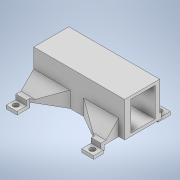
# Autodesk Inventor part: U2D2 Plate v2
Saved by Autodesk Inventor 2022 (Build 260153000, 153)
## iProperties
Created: 2021-09-20
Part Number: U2D2 Plate v2
Material: Generic
Document SubType Name: Modeling
Designer: kylem
Density: 1 g/cm^3
Appearance: Default
Author: kylem
Autodesk Inventor part; units mm, degrees
note: some values were not read from the file. Chosen so that the rebuilt part matches the saved one: edges of "Chamfer23".
ref_plane "YZ Plane" through (0, 0, 0) normal (1, 0, 0) x (0, 1, 0)
sketch "Sketch1" plane through (0, 0, 0) normal (0, 1, 0) x (-1, 0, 0)
  line L0 (0, 0) -> (3, 0)
  line L1 (3, 0) -> (3, -3)
  line L2 (0, 0) -> (-48.04, 0)
  line L3 (-48.04, 0) -> (-54, 0)
  line L4 (3, -3) -> (-54, -3)
  line L5 (-54, -3) -> (-54, 45)
  line L6 (-54, 45) -> (3, 45)
  line L7 (3, 45) -> (3, -3)
  line L8 (3, 21) -> (6.1215, 21)
  circle A0 centre (0, 0) radius 1.65
  circle A1 centre (-48.04, 0) radius 1.65
  line L9 (0, 42) -> (-48.04, 42)
  circle A2 centre (0, 42) radius 1.65
  circle A3 centre (-48.04, 42) radius 1.65
  line L10 (-54, -3) -> (-54, 8.785)
  line L11 (-54, 8.785) -> (-9.9, 8.785)
  line L12 (-9.9, 8.785) -> (-9.9, 23.785)
  line L13 (-9.9, 23.785) -> (-54, 23.785)
  dimension "d0" = 3
  dimension "d1" = 3
  dimension "d2" = 48.04
  dimension "d3" = 5.96
  dimension "d4" = 48
  dimension "d5" = 3.3
  dimension "d6" = 3.3
  dimension "d7" = 11.785
  dimension "d8" = 44.1
  dimension "d9" = 15
  constraints: 28 end point, 5 perpendicular, 4 centre point, 4 coincident, 4 horizontal, 4 symmetric about line, 3 point on line, 2 parallel, 1 midpoint, 2 other
  measures "d0" distance of L0.start L0.end
  measures "d1" distance of L0.end L1.end
  measures "d2" distance of L0.start L2.end
  measures "d3" distance of L2.end L3.end
  measures "d4" distance of L4.end L5.end
  measures "d5" diameter of A0
  measures "d6" diameter of A1
  measures "d7" distance of L4.end L10.end
  measures "d8" distance of L10.end L11.end
  measures "d9" distance of L11.end L12.end
extrude "Extrusion1" add sketch "Sketch1" along normal blind 2 contours A0 L2 A1 L3 L5 L11 L12 L13 L6 L7 L0 | L0 L1 L4 L5 L3 A1 L2 A0
sketch "Sketch2" plane through (0, 0, 0) normal (0, -1, 0) x (1, 0, 0)
  line L0 (-3, -3) -> (-3, 45) projected
  line L1 (-3, -3) -> (-3, 5)
  line L2 (54, 8.785) -> (54, -3) projected
  line L3 (9.9, 8.785) -> (54, 8.785) projected
  line L4 (54, 8.785) -> (54, 4.785)
  line L5 (54, 8.785) -> (54, -3) projected
  line L6 (54, 23.785) -> (54, 27.785)
  line L7 (54, 45) -> (54, 23.785) projected
  line L8 (54, 27.785) -> (-3, 27.785)
  line L9 (-3, 5) -> (-3, 27.785)
  line L10 (9.9, 8.785) -> (54, 8.785) projected
  line L11 (54, 8.785) -> (9.9, 8.785)
  line L12 (9.9, 23.785) -> (9.9, 8.785) projected
  line L13 (9.9, 8.785) -> (9.9, 23.785)
  line L14 (9.9, 23.785) -> (54, 23.785)
  line L15 (-3, 5) -> (-3, 27.785)
  line L16 (-3, 27.785) -> (54, 27.785)
  line L17 (54, 27.785) -> (54, 4.785)
  line L18 (54, 4.785) -> (-3, 4.785)
  line L19 (-3, 4.785) -> (-3, 27.785)
  point P0 (0, 0)
  point P1 (-3, 4.785)
  dimension "d12" = 8
  dimension "d13" = 4
  dimension "d14" = 4
  constraints: 26 end point, 4 collinear, 4 point on line, 3 perpendicular, 2 parallel, 1 horizontal
  measures "d12" distance of L0.start L1.end
  measures "d13" distance of L2.start L4.end
  measures "d14" distance of L6.start L6.end
ref_plane "Work Plane1" through (0, -7, 0) normal (0, -1, 0) x (1, 0, 0)
sketch "Sketch4" plane through (54, 0, -3) normal (1, 0, 0) x (0, 0, -1)
  line L0 (-7.785, 0) -> (-7.785, -7) projected
  line L1 (-7.785, 0) -> (-7.785, 2)
  line L2 (0, 2) -> (-48, 2) projected
  line L3 (-7.785, 2) -> (-7.785, 15)
  line L4 (-30.785, 0) -> (-30.785, -7) projected
  line L5 (-30.785, 0) -> (-30.785, 15)
  line L6 (-7.785, 15) -> (-30.785, 15)
  line L7 (-26.785, -5) -> (-11.785, -5) projected
  line L8 (-11.785, 0) -> (-11.785, 2) projected
  line L9 (-11.785, -5) -> (-11.785, 2)
  line L10 (-11.785, 2) -> (-11.785, 13)
  line L11 (-26.785, 0) -> (-26.785, 2) projected
  line L12 (-26.785, 2) -> (-26.785, 13)
  line L13 (-26.785, 13) -> (-11.785, 13)
  point P0 (-3, 0)
  point P1 (-30.785, 2)
  dimension "d19" = 13
  dimension "d20" = 15
  dimension "d21" = 11
  dimension "d22" = 11
  constraints: 16 end point, 3 point on line, 2 collinear, 2 vertical
  measures "d19" distance of L1.end L3.end
  measures "d20" distance of L4.start L5.end
  measures "d21" distance of L8.end L10.end
  measures "d22" distance of L11.end L12.end
extrude "Extrusion5" add sketch "Sketch2" along normal blind 7 contours L0 L8 L6 L14 L12 L3 L2 L18
sketch "Sketch5" plane through (0, -7, 0) normal (0, -1, 0) x (1, 0, 0)
  line L0 (9.9, 23.785) -> (54, 23.785) projected
  line L1 (54, 23.785) -> (9.9, 23.785)
  line L2 (9.9, 23.785) -> (9.9, 8.785)
  line L3 (9.9, 8.785) -> (54, 8.785)
  line L4 (54, 8.785) -> (54, 23.785)
  point P0 (0, 0)
  constraints: 8 end point, 2 parallel, 1 horizontal, 1 perpendicular
extrude "Extrusion6" add sketch "Sketch5" against normal blind 2
extrude "Extrusion7" add sketch "Sketch4" against normal blind 44.1 contours L2 L10 L13 L12 L5 L6 L3
sketch "Sketch6" plane through (9.9, 0, -3) normal (-1, 0, 0) x (0, 0, 1)
  line L0 (7.785, 15) -> (7.785, 2) projected
  line L1 (48, 2) -> (30.785, 2) projected
  line L2 (7.785, 15) -> (30.785, 15)
  line L3 (30.785, 15) -> (30.785, 2)
  line L4 (30.785, 2) -> (7.785, 2)
  line L5 (7.785, 2) -> (7.785, 15)
  point P0 (3, 0)
  constraints: 8 end point, 2 parallel, 1 horizontal, 1 perpendicular
extrude "Extrusion8" add sketch "Sketch6" along normal blind 12.9
sketch "Sketch8" plane through (9.9, -5, 8.785) normal (0, 0, 1) x (1, 0, 0)
  line L0 (44.1, 0) -> (44.1, 18) projected
  line L1 (44.1, 0) -> (18.5, 0)
  line L2 (0, 0) -> (44.1, 0) projected
  line L3 (18.5, 0) -> (5.5, 0)
  line L4 (5.5, 0) -> (5.5, 1)
  line L5 (-12.9, 5) -> (44.1, 5) projected
  line L6 (5.5, 1) -> (14.6, 1)
  line L7 (44.1, -2) -> (-12.9, -2) projected
  line L8 (44.1, 18) -> (0, 18) projected
  line L9 (14.6, -2) -> (36.6, -2) construction
  line L10 (5.5, 1) -> (5.5, 18)
  line L11 (5.5, 18) -> (14.6, 18)
  line L12 (44.1, 18) -> (0, 18) projected
  line L13 (5.5, 1) -> (5.5, 17)
  line L14 (5.5, 17) -> (14.6, 17)
  line L15 (5.5, 17) -> (18.5, 17)
  line L16 (18.5, 17) -> (18.5, 1)
  line L17 (18.5, 1) -> (5.5, 1)
  point P0 (-9.9, 5)
  point P1 (5.5, 5)
  point P2 (14.6, 1)
  dimension "d33" = 25.6
  dimension "d34" = 13
  dimension "d35" = 1
  dimension "d39" = 16
  dimension "d42" = 13
  constraints: 24 end point, 7 point on line, 3 perpendicular, 1 collinear, 1 horizontal
  measures "d33" distance of L0.start L1.end
  measures "d34" distance of L1.end L3.end
  measures "d35" distance of L3.end L4.end
  measures "d39" distance of L4.end L13.end
  measures "d42" distance of L13.end L15.end
extrude "Extrusion10" cut sketch "Sketch8" against normal blind 12.9 contours L16 L17 L6 L10 L5 | L5 L10 L14 L15 L16
sketch "Sketch11" plane through (0, 2, 0) normal (0, 1, 0) x (1, 0, 0)
  circle A0 centre (48.04, 0) radius 1.65 projected
  circle A1 centre (0, 0) radius 1.65 projected
  line L0 (48.04, 0) -> (0, 0)
  line L1 (24.02, 0) -> (24.02, 5.2317)
  line L2 (24.02, 0) -> (10.02, 0)
  line L3 (10.02, 0) -> (38.02, 0)
  line L4 (38.02, 0) -> (38.02, 7.5339)
  line L5 (54, -4.785) -> (-3, -4.785) projected
  line L6 (38.02, 7.5339) -> (10.02, 7.5339)
  line L7 (10.02, 7.5339) -> (10.02, -4.785)
  line L8 (10.02, -4.785) -> (38.02, -4.785)
  line L9 (38.02, -4.785) -> (38.02, 7.5339)
  dimension "d74" = 14
  dimension "d75" = 28
  constraints: 18 end point, 3 point on line, 2 horizontal, 2 parallel, 2 perpendicular, 1 midpoint, 1 vertical
  measures "d74" distance of L1.start L2.end
  measures "d75" distance of L2.end L3.end
extrude "Extrusion12" cut sketch "Sketch11" against normal blind 10 contours L9 L5 L7 L0 | L0 L7 L6 L4
chamfer "Chamfer9" distance 7.785 angle 45 2 edges at (38.02, 1, -3) (10.02, 1, -3)
sketch "Sketch12" plane through (54, 13, 8.785) normal (0, -1, 0) x (1, 0, 0)
  line L0 (0, 0) -> (-44.1, 0) projected
  line L1 (-44.1, 0) -> (-44.1, 15) projected
  line L2 (0, 0) -> (-44.1, 0)
  line L3 (-44.1, 0) -> (-44.1, 15)
  line L4 (-44.1, 15) -> (0, 15)
  line L5 (0, 15) -> (0, 0)
  point P0 (-54, -8.785)
  constraints: 8 end point, 2 parallel, 1 horizontal, 1 perpendicular
extrude "Extrusion13" cut sketch "Sketch12" against normal blind 0.17
sketch "Sketch13" plane through (0, -5, 0) normal (0, 1, 0) x (1, 0, 0)
  line L0 (54, -23.785) -> (9.9, -23.785) projected
  line L1 (9.9, -8.785) -> (54, -8.785)
  line L2 (54, -8.785) -> (54, -23.785)
  line L3 (54, -23.785) -> (9.9, -23.785)
  line L4 (9.9, -23.785) -> (9.9, -8.785)
  point P0 (0, 0)
  constraints: 8 end point, 2 parallel, 1 horizontal, 1 perpendicular
extrude "Extrusion14" cut sketch "Sketch13" against normal blind 0.17
sketch "Sketch14" plane through (54, 13.17, 23.785) normal (0, 0, -1) x (-1, 0, 0)
  line L0 (44.1, -18.34) -> (44.1, 0) projected
  line L1 (0, -18.34) -> (44.1, -18.34) projected
  line L2 (44.1, 0) -> (0, 0)
  line L3 (0, 0) -> (0, -18.34)
  line L4 (0, -18.34) -> (44.1, -18.34)
  line L5 (44.1, -18.34) -> (44.1, 0)
  point P0 (54, -13.17)
  constraints: 8 end point, 2 parallel, 1 horizontal, 1 perpendicular
extrude "Extrusion15" cut sketch "Sketch14" against normal blind 0.07
sketch "Sketch15" plane through (9.9, 13.17, 8.785) normal (0, 0, 1) x (1, 0, 0)
  line L0 (44.1, 0) -> (0, 0) projected
  line L1 (44.1, 0) -> (44.1, -18.34) projected
  line L2 (0, 0) -> (44.1, 0)
  line L3 (44.1, 0) -> (44.1, -18.34)
  line L4 (44.1, -18.34) -> (0, -18.34)
  line L5 (0, -18.34) -> (0, 0)
  point P0 (-9.9, -13.17)
  constraints: 8 end point, 2 parallel, 1 horizontal, 1 perpendicular
extrude "Extrusion16" cut sketch "Sketch15" against normal blind 0.07
ref_plane "Work Plane2" through (0, -10, 0) normal (0, -1, 0) x (1, 0, 0)
sketch "Sketch16" plane through (0, -10, 0) normal (0, -1, 0) x (1, 0, 0)
  circle A0 centre (0, 42) radius 1.65 projected
  circle A1 centre (0, 42) radius 1.65
  line L0 (0, 42) -> (0, 45)
  line L1 (-3, 45) -> (54, 45) projected
  line L2 (0, 45) -> (3.75, 45)
  line L3 (3.75, 45) -> (3.75, 39)
  line L4 (3.75, 39) -> (-3.75, 39)
  line L5 (-3.75, 39) -> (-3.75, 45)
  line L6 (-3.75, 45) -> (3.75, 45)
  circle A2 centre (48.04, 42) radius 1.65 projected
  line L7 (0, 42) -> (48.04, 42)
  line L8 (24.02, 42) -> (24.02, 49.286)
  circle A3 centre (48.04, 42) radius 1.65
  circle A4 centre (48.04, 42) radius 1.65
  line L9 (48.04, 42) -> (48.04, 45)
  line L10 (51.04, 45) -> (-5.96, 45)
  line L11 (48.04, 45) -> (44.29, 45)
  line L12 (44.29, 45) -> (44.29, 39)
  line L13 (44.29, 39) -> (51.79, 39)
  line L14 (51.79, 39) -> (51.79, 45)
  line L15 (51.79, 45) -> (44.29, 45)
  line L16 (48.04, 42) -> (0, 42)
  line L17 (0, 42) -> (0, 0)
  line L18 (0, 21) -> (5.7249, 21)
  circle A5 centre (0, 0) radius 1.65
  circle A6 centre (0, 0) radius 1.65
  line L19 (0, 0) -> (0, -3)
  line L20 (-3, -3) -> (54, -3)
  line L21 (0, -3) -> (3.75, -3)
  line L22 (3.75, -3) -> (3.75, 3)
  line L23 (3.75, 3) -> (-3.75, 3)
  line L24 (-3.75, 3) -> (-3.75, -3)
  line L25 (-3.75, -3) -> (3.75, -3)
  circle A7 centre (48.04, 0) radius 1.65
  line L26 (0, 0) -> (48.04, 0)
  line L27 (24.02, 0) -> (24.02, -7.286)
  circle A8 centre (48.04, 0) radius 1.65
  circle A9 centre (48.04, 0) radius 1.65
  line L28 (48.04, 0) -> (48.04, -3)
  line L29 (51.04, -3) -> (-5.96, -3)
  line L30 (48.04, -3) -> (44.29, -3)
  line L31 (44.29, -3) -> (44.29, 3)
  line L32 (44.29, 3) -> (51.79, 3)
  line L33 (51.79, 3) -> (51.79, -3)
  line L34 (51.79, -3) -> (44.29, -3)
  line L35 (48.04, 0) -> (0, 0)
  line L36 (0, 0) -> (0, 42)
  line L37 (44.29, 39) -> (50.29, 39)
  line L38 (50.29, 39) -> (50.29, 37)
  line L39 (50.29, 37) -> (44.29, 37)
  line L40 (44.29, 37) -> (44.29, 39)
  line L41 (3.75, 39) -> (-3.75, 39)
  line L42 (-3.75, 39) -> (-3.75, 37)
  line L43 (-3.75, 37) -> (3.75, 37)
  line L44 (3.75, 37) -> (3.75, 39)
  line L45 (3.75, 3) -> (-3.75, 3)
  line L46 (-3.75, 3) -> (-3.75, 4.785)
  line L47 (-3.75, 4.785) -> (3.75, 4.785)
  line L48 (3.75, 4.785) -> (3.75, 3)
  line L49 (-3, 4.785) -> (54, 4.785) projected
  line L50 (51.79, 3) -> (44.29, 3)
  line L51 (44.29, 3) -> (44.29, 4.785)
  line L52 (44.29, 4.785) -> (51.79, 4.785)
  line L53 (51.79, 4.785) -> (51.79, 3)
  dimension "d102" = 3.75
  dimension "d103" = 6
  dimension "d104" = 7.5
  dimension "d107" = 6
  dimension "d108" = 2
  dimension "d109" = 2
  constraints: 104 end point, 33 symmetric about line, 9 perpendicular, 8 centre point, 8 parallel, 7 point on line, 6 horizontal, 4 coincident, 2 midpoint, 2 vertical, 1 collinear, 7 other
  measures "d102" distance of L0.end L2.end
  measures "d103" distance of L2.end L3.end
  measures "d104" distance of L3.end L4.end
  measures "d107" distance of L38.end L39.end
  measures "d108" distance of L37.end L38.end
  measures "d109" distance of L42.end L41.end
extrude "Extrusion18" add sketch "Sketch16" against normal blind 2 contours L7 L3 L4 L17 A0 | A0 L0 L1 L3 L7 | A0 L17 L4 L5 L6 L1 L0 | L17 L43 L42 L4 | L4 L44 L43 L17 | L12 L1 L9 A2 L7 | L7 A2 L9 L1 L14 L13 L12 | L13 L38 L39 L40 | L47 L48 L23 L17 | L17 L23 L46 L47 | L23 L22 L26 A5 L17 | L17 A5 L19 L20 L25 L24 L23 | L49 L53 L32 L51 | L26 L22 L20 L19 A5 | L32 L33 L20 L28 A7 L26 L31 | L26 A7 L28 L20 L31
sketch "Sketch19" plane through (0, -10, 0) normal (0, -1, 0) x (1, 0, 0)
  circle A0 centre (0, 42) radius 1.65
  circle A1 centre (0, 42) radius 1.65
  line L0 (0, 42) -> (0, 45)
  line L1 (-3, 45) -> (54, 45)
  line L2 (0, 45) -> (3.75, 45)
  line L3 (3.75, 45) -> (3.75, 39)
  line L4 (3.75, 39) -> (-3.75, 39)
  line L5 (-3.75, 39) -> (-3.75, 45)
  line L6 (-3.75, 45) -> (3.75, 45)
  circle A2 centre (48.04, 42) radius 1.65
  line L7 (0, 42) -> (48.04, 42)
  line L8 (24.02, 42) -> (24.02, 49.286)
  circle A3 centre (48.04, 42) radius 1.65
  circle A4 centre (48.04, 42) radius 1.65
  line L9 (48.04, 42) -> (48.04, 45)
  line L10 (51.04, 45) -> (-5.96, 45)
  line L11 (48.04, 45) -> (44.29, 45)
  line L12 (44.29, 45) -> (44.29, 39)
  line L13 (44.29, 39) -> (51.79, 39)
  line L14 (51.79, 39) -> (51.79, 45)
  line L15 (51.79, 45) -> (44.29, 45)
  line L16 (48.04, 42) -> (0, 42)
  line L17 (0, 42) -> (0, 0)
  line L18 (0, 21) -> (5.7249, 21)
  circle A5 centre (0, 0) radius 1.65
  circle A6 centre (0, 0) radius 1.65
  line L19 (0, 0) -> (0, -3)
  line L20 (0, -3) -> (3.75, -3)
  line L21 (3.75, -3) -> (3.75, 3)
  line L22 (3.75, 3) -> (-3.75, 3)
  line L23 (-3.75, 3) -> (-3.75, -3)
  line L24 (-3.75, -3) -> (3.75, -3)
  line L25 (0, 0) -> (0, 42)
  line L26 (-3, -3) -> (54, -3)
  line L27 (24.02, 0) -> (24.02, -7.286)
  line L28 (44.29, -3) -> (44.29, 3)
  line L29 (48.04, -3) -> (44.29, -3)
  line L30 (0, 0) -> (48.04, 0)
  line L31 (48.04, 0) -> (48.04, -3)
  line L32 (48.04, 0) -> (0, 0)
  circle A7 centre (48.04, 0) radius 1.65
  circle A8 centre (48.04, 0) radius 1.65
  circle A9 centre (48.04, 0) radius 1.65
  line L33 (44.29, 3) -> (51.79, 3)
  line L34 (51.79, 3) -> (51.79, -3)
  line L35 (51.79, -3) -> (44.29, -3)
  line L36 (51.04, -3) -> (-5.96, -3)
  line L37 (44.29, 39) -> (50.29, 39)
  line L38 (50.29, 39) -> (50.29, 37)
  line L39 (50.29, 37) -> (44.29, 37)
  line L40 (44.29, 37) -> (44.29, 39)
  line L41 (3.75, 39) -> (-3.75, 39)
  line L42 (-3.75, 39) -> (-3.75, 37)
  line L43 (-3.75, 37) -> (3.75, 37)
  line L44 (3.75, 37) -> (3.75, 39)
  line L45 (3.75, 3) -> (-3.75, 3)
  line L46 (-3.75, 3) -> (-3.75, 4.785)
  line L47 (-3.75, 4.785) -> (3.75, 4.785)
  line L48 (3.75, 4.785) -> (3.75, 3)
  line L49 (-3, 4.785) -> (54, 4.785)
  line L50 (51.79, 3) -> (44.29, 3)
  line L51 (44.29, 3) -> (44.29, 4.785)
  line L52 (44.29, 4.785) -> (51.79, 4.785)
  line L53 (51.79, 4.785) -> (51.79, 3)
  dimension "d118" = 3.75
  dimension "d119" = 6
  dimension "d120" = 7.5
  dimension "d121" = 6
  dimension "d122" = 2
  dimension "d123" = 2
  constraints: 108 end point, 33 symmetric about line, 10 centre point, 9 perpendicular, 8 parallel, 7 point on line, 6 horizontal, 4 coincident, 2 midpoint, 2 vertical, 1 collinear, 7 other
  measures "d118" distance of L0.end L2.end
  measures "d119" distance of L2.end L3.end
  measures "d120" distance of L3.end L4.end
  measures "d121" distance of L38.end L39.end
  measures "d122" distance of L37.end L38.end
  measures "d123" distance of L42.end L41.end
extrude "Extrusion19" add sketch "Sketch19" against normal blind 5 contours L17 L43 L42 L4 | L4 L44 L43 L17 | L13 L38 L39 L40 | L47 L48 L22 L17 | L17 L22 L46 L47 | L49 L53 L33 L51
sketch "Sketch21" plane through (-3.75, -10, 37) normal (-1, 0, 0) x (0, 0, 1)
  line L0 (10.7481, 37.9604) -> (-46.1499, 37.9604)
  line L1 (-46.1499, 37.9604) -> (-46.1499, -17.1165)
  line L2 (-46.1499, -17.1165) -> (10.7481, -17.1165)
  line L3 (10.7481, -17.1165) -> (10.7481, 37.9604)
  point P0 (-37, 10)
  constraints: 8 end point, 2 parallel, 1 horizontal, 1 perpendicular
extrude "Extrusion20" cut sketch "Sketch21" against normal blind 0.75
sketch "Sketch22" plane through (54, -7, 4.785) normal (0, 0, -1) x (-1, 0, 0)
  line L0 (-3.9524, 17.9954) -> (64.8969, 17.9954)
  line L1 (64.8969, 17.9954) -> (64.8969, 4.1625)
  line L2 (64.8969, 4.1625) -> (-3.9524, 4.1625)
  line L3 (-3.9524, 4.1625) -> (-3.9524, 17.9954)
  point P0 (54, 7)
  constraints: 8 end point, 2 parallel, 1 horizontal, 1 perpendicular
extrude "Extrusion21" cut sketch "Sketch22" along normal blind 10
sketch "Sketch23" plane through (54, 2, 27.785) normal (0, 0, 1) x (1, 0, 0)
  line L0 (-60.01, 3.5962) -> (0.9573, 3.5962)
  line L1 (0.9573, 3.5962) -> (0.9573, -3.8917)
  line L2 (0.9573, -3.8917) -> (-60.01, -3.8917)
  line L3 (-60.01, -3.8917) -> (-60.01, 3.5962)
  point P0 (-54, -2)
  constraints: 8 end point, 2 parallel, 1 horizontal, 1 perpendicular
extrude "Extrusion22" cut sketch "Sketch23" along normal blind 20
sketch "Sketch24" plane through (0, -5, 0) normal (0, 1, 0) x (1, 0, 0)
  line L0 (54, -27.785) -> (-3, -27.785) projected
  line L1 (-3, -39) -> (3.75, -39)
  line L2 (3.75, -39) -> (3.75, -27.785)
  line L3 (3.75, -27.785) -> (-3, -27.785)
  line L4 (-3, -27.785) -> (-3, -39)
  line L5 (50.29, -37) -> (50.29, -39) projected
  line L6 (50.29, -39) -> (44.29, -39)
  line L7 (44.29, -39) -> (44.29, -27.785)
  line L8 (44.29, -27.785) -> (50.29, -27.785)
  line L9 (50.29, -27.785) -> (50.29, -39)
  point P0 (0, 0)
  dimension "d132" = 6.75
  dimension "d133" = 6
  constraints: 16 end point, 4 parallel, 2 horizontal, 2 perpendicular, 2 point on line
  measures "d132" distance of L3.end L2.end
  measures "d133" distance of L7.end L8.end
extrude "Extrusion23" add sketch "Sketch24" against normal blind 2
chamfer "Chamfer17" distance 1.75 angle 45 2 edges at (0.375, -5, 4.785) (48.04, -5, 4.785)
chamfer "Chamfer20" distance 8 angle 45 2 edges at (0.375, -5, 27.785) (47.29, -5, 27.785)
chamfer "Chamfer21" distance 16 angle 30 2 edges at (44.29, -6, 27.785) (44.29, -1, 27.785) measured on face at (31.7633, 11, 27.785)
chamfer "Chamfer22" distance 16 angle 30 2 edges at (3.75, -6, 27.785) (3.75, -1, 27.785) measured on face at (26.43, 11, 27.785)
chamfer "Chamfer23" distance 3.091 angle 30 1 edges at (44.29, -6, 4.785)
chamfer "Chamfer24" distance 3.091 angle 30 1 edges at (3.75, -5.125, 4.785) measured on face at (41.1997, 7.9167, 4.785)
sketch "Sketch25" plane through (54, -7, 4.785) normal (0, 0, -1) x (-1, 0, 0)
  line L0 (38.6, 19) -> (38.6, 3) projected
  line L1 (38.6, 19) -> (41.6, 19)
  line L2 (41.6, 19) -> (41.6, 3)
  line L3 (41.6, 3) -> (38.6, 3)
  line L4 (38.6, 3) -> (38.6, 19)
  point P0 (54, 7)
  point P1 (38.6, 3)
  dimension "d169" = 3
  constraints: 8 end point, 2 parallel, 1 horizontal, 1 perpendicular
  measures "d169" distance of L2.end L3.end
extrude "Extrusion24" cut sketch "Sketch25" against normal blind 5
sketch "Sketch26" plane through (9.9, -5.17, 23.855) normal (1, 0, 0) x (0, 0, -1)
  line L0 (15.14, 0) -> (0, 0) projected
  line L1 (0, 18.34) -> (15.14, 18.34) projected
  line L2 (0, 0) -> (15.14, 0)
  line L3 (15.14, 0) -> (15.14, 18.34)
  line L4 (15.14, 18.34) -> (0, 18.34)
  line L5 (0, 18.34) -> (0, 0)
  point P0 (23.855, 5.17)
  constraints: 8 end point, 2 parallel, 1 horizontal, 1 perpendicular
extrude "Extrusion25" add sketch "Sketch26" along normal blind 0.75
sketch "Sketch27" plane through (10.65, -5.17, 23.855) normal (1, 0, 0) x (0, 0, -1)
  line L0 (15.14, 0) -> (0, 0) projected
  line L1 (0, 0) -> (15.14, 0)
  line L2 (0, 18.34) -> (15.14, 18.34) projected
  line L3 (15.14, 0) -> (15.14, 18.34)
  line L4 (15.14, 18.34) -> (15.14, 0)
  line L5 (15.14, 1.17) -> (15.14, 17.17) projected
  line L6 (15.14, 9.17) -> (0, 9.17)
  line L7 (0, 0) -> (0, 18.34) projected
  line L8 (7.57, 0) -> (7.57, 18.34)
  circle A0 centre (7.57, 9.17) radius 3
  point P0 (23.855, 5.17)
  dimension "d174" = 6
  constraints: 10 end point, 4 midpoint, 1 centre point, 1 collinear, 1 perpendicular, 1 vertical
  measures "d174" diameter of A0
extrude "Extrusion26" cut sketch "Sketch27" against normal blind 30 contours A0 L6 L8 | L8 L6 A0 | L8 A0 L6 | L6 A0 L8
sketch "Sketch28" plane through (54, -7, 4.785) normal (0, 0, -1) x (-1, 0, 0)
  line L0 (0, 0) -> (0, 22) projected
  line L1 (57, 10) -> (57, 2) projected
  line L2 (0, 22) -> (57, 22)
  line L3 (57, 22) -> (57, 3.75)
  line L4 (57, 3.75) -> (0, 3.75)
  line L5 (0, 3.75) -> (0, 22)
  line L6 (2.21, 3.75) -> (12.801, 3.75) projected
  line L7 (50.25, 0) -> (47.159, 0) projected
  line L8 (12.801, 3.75) -> (47.159, 3.75)
  line L9 (47.159, 3.75) -> (47.159, 0)
  line L10 (47.159, 0) -> (12.801, 0)
  line L11 (12.801, 0) -> (12.801, 3.75)
  point P0 (54, 7)
  dimension "d177" = 18.25
  constraints: 16 end point, 4 parallel, 2 horizontal, 2 perpendicular, 1 point on line
  measures "d177" distance of L2.end L3.end
extrude "Extrusion27" cut sketch "Sketch28" against normal blind 1
chamfer "Chamfer25" distance 1 angle 45 2 edges at (41.199, -5.125, 5.785) (6.841, -5.125, 5.785)
sketch "Sketch29" plane through (10.65, -5.17, 23.855) normal (1, 0, 0) x (0, 0, -1)
  line L0 (0, 0) -> (0, 18.34) projected
  line L1 (0, 18.34) -> (15.14, 18.34) projected
  line L2 (0, 0) -> (15.14, 0)
  line L3 (15.14, 0) -> (15.14, 18.34)
  line L4 (15.14, 18.34) -> (0, 18.34)
  line L5 (0, 18.34) -> (0, 0)
  point P0 (23.855, 5.17)
  constraints: 8 end point, 2 parallel, 1 horizontal, 1 perpendicular
extrude "Extrusion28" cut sketch "Sketch29" against normal blind 1
sketch "Sketch30" plane through (54, -7, 5.785) normal (0, 0, -1) x (-1, 0, 0)
  line L0 (41.6, 3) -> (25.6, 3) projected
  line L1 (25.6, 3) -> (23.6, 3)
  line L2 (23.6, 3) -> (23.6, 19)
  line L3 (23.6, 19) -> (25.6, 19)
  line L4 (25.6, 19) -> (25.6, 3)
  point P0 (54, 7)
  dimension "d185" = 2
  dimension "d186" = 16
  constraints: 8 end point, 2 parallel, 1 horizontal, 1 perpendicular
  measures "d185" distance of L2.end L3.end
  measures "d186" distance of L1.end L2.end
extrude "Extrusion29" cut sketch "Sketch30" against normal blind 5
body "Solid1"
